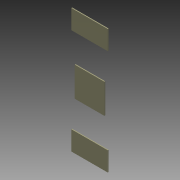
# Autodesk Inventor part: leakage
Saved by Autodesk Inventor 2015 (Build 190159000, 159)
## iProperties
Created: 2014-10-08
Part Number: leakage
Material: Polypropylene
Document SubType Name: Modeling
Designer: Adam
Density: 0.899 g/cm^3
Appearance: Smooth - Ash
Author: Adam
Autodesk Inventor part; units mm, degrees
ref_plane "YZ Plane" through (0, 0, 0) normal (1, 0, 0) x (0, 1, 0)
ref_plane "XZ Plane" through (0, 0, 0) normal (0, 1, 0) x (-1, 0, 0)
ref_plane "XY Plane" through (0, 0, 0) normal (0, 0, 1) x (1, 0, 0)
sketch "Sketch1" plane through (0, 0, 0) normal (0, 0, 1) x (1, 0, 0)
  line L0 (0, 0) -> (0, -4.565) projected
  line L1 (0, -4.565) -> (9.53, -4.565) projected
  line L2 (9.53, 0) -> (9.53, -4.565) projected
  line L3 (0, 0) -> (9.53, 0) projected
  line L4 (0, -12.7) -> (0, -22.23) projected
  line L5 (0, -22.23) -> (9.53, -22.23) projected
  line L6 (9.53, -12.7) -> (9.53, -22.23) projected
  line L7 (0, -12.7) -> (9.53, -12.7) projected
  line L8 (0, -30.365) -> (0, -34.93) projected
  line L9 (0, -34.93) -> (9.53, -34.93) projected
  line L10 (9.53, -30.365) -> (9.53, -34.93) projected
  line L11 (0, -30.365) -> (9.53, -30.365) projected
  line L12 (10.03, 0.5) -> (-0.5, 0.5)
  line L13 (-0.5, 0.5) -> (-0.5, -5.065)
  line L14 (-0.5, -5.065) -> (10.03, -5.065)
  line L15 (10.03, -5.065) -> (10.03, 0.5)
  line L16 (9.03, -13.2) -> (0.5, -13.2)
  line L17 (0.5, -13.2) -> (0.5, -21.73)
  line L18 (0.5, -21.73) -> (9.03, -21.73)
  line L19 (9.03, -21.73) -> (9.03, -13.2)
  line L20 (10.03, -29.865) -> (-0.5, -29.865)
  line L21 (-0.5, -29.865) -> (-0.5, -35.43)
  line L22 (-0.5, -35.43) -> (10.03, -35.43)
  line L23 (10.03, -35.43) -> (10.03, -29.865)
  dimension "d0" = 0.5
  dimension "d1" = 0.5
  dimension "d2" = 0.5
  dimension "d3" = 0.5
  dimension "d4" = 0.5
  dimension "d5" = 0.5
  dimension "d6" = 0.5
  dimension "d7" = 0.5
  dimension "d8" = 0.5
  dimension "d9" = 0.5
  constraints: 24 end point, 6 parallel, 3 horizontal, 3 perpendicular, 1 collinear, 1 point on line
  measures "d0" distance between parallel lines of L9 L22
  measures "d1" distance between parallel lines of L11 L20
  measures "d2" distance between parallel lines of L10 L23
  measures "d3" distance between parallel lines of L21 L8
  measures "d4" distance between parallel lines of L4 L17
  measures "d5" distance between parallel lines of L7 L16
  measures "d6" distance between parallel lines of L19 L6
  measures "d7" distance between parallel lines of L5 L18
  measures "d8" distance between parallel lines of L1 L14
  measures "d9" distance between parallel lines of L12 L3
extrude "Extrusion1" add sketch "Sketch1" along normal blind 0.25 contours L3 L2 L1 L0 | L11 L10 L9 L8 | L15 L14 L13 L12 | L19 L18 L17 L16 | L23 L22 L21 L20
equation "\"d1\" = d0"
equation "\"d2\" = d0"
equation "\"d3\" = d0"
equation "\"d4\" = d0"
equation "\"d5\" = d0"
equation "\"d6\" = d0"
equation "\"d7\" = d0"
equation "\"d8\" = d0"
equation "\"d9\" = d0"
body "Solid1"
